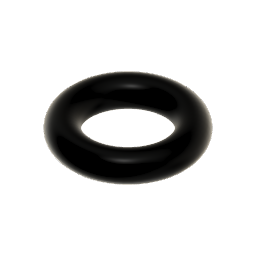
Rubber_9mm (Autodesk Fusion 360 design; units mm, degrees)
Autodesk Fusion 360 part; units mm, degrees
sketch "Sketch1" plane through (0, 0, 0) normal (0, 0, 1) x (1, 0, 0)
  circle A0 centre (0, 0) radius 4.5
  circle A1 centre (0, 0) radius 2.5
  dimension "d1" = 9
  dimension "d2" = 5
  constraint coincident A0.centre A1.centre
  measures "d1" diameter of A0
  measures "d2" diameter of A1
extrude "Extrude1" add sketch "Sketch1" along normal blind 2
fillet "Fillet1" radius 1 4 edges at (-4.1955, -1.6273, 2) (-4.1955, -1.6273, 0) (-2.3308, 0.904, 2) (-2.3308, 0.904, 0)
equation "d1 = outerDiameter"
equation "d2 = innerDiameter"
equation "d3 = height"
equation "d6 = height / 2"
equation "outerDiameter = 9 mm"
equation "innerDiameter = 5 mm"
equation "height = 2 mm"
named bodies: "Rubber_9mm"
